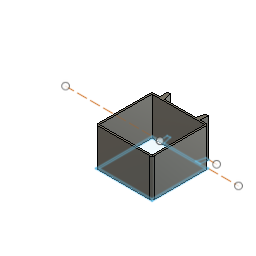
VoltmeterEnclosure (Autodesk Fusion 360 design; units mm, degrees)
Autodesk Fusion 360 part; units mm, degrees
note: some values were not read from the file. Set by a fixed rule: which sketch regions a step uses.
other "Base Mesh Feature1"
sketch "Sketch2" plane through (0, 0, 0) normal (0, 1, 0) x (1, 0, 0)
  line L0 (38.15, -96.15) -> (-38.15, -96.15)
  line L1 (-38.15, -96.15) -> (-38.15, -19.85)
  line L2 (-38.15, -19.85) -> (38.15, -19.85)
  line L3 (38.15, -19.85) -> (38.15, -96.15)
  line L4 (40.65, -98.65) -> (-40.65, -98.65)
  line L5 (-40.65, -98.65) -> (-40.65, -17.35)
  line L6 (-40.65, -17.35) -> (40.65, -17.35)
  line L7 (40.65, -17.35) -> (40.65, -98.65)
  line L8 (28.7422, -17.35) -> (22.7422, -17.35)
  line L9 (22.7422, -17.35) -> (25.6453, -5.7065)
  line L10 (22.7422, -17.35) -> (84.5269, -17.35) construction
  line L11 (30.0696, -6) -> (29.0766, -17.35)
  line L12 (30.0696, -6) -> (41.5439, -6) construction
  line L13 (28.7422, -17.35) -> (22.7422, -17.35)
  line L14 (30.0696, -6) -> (25.6453, -5.7065)
  line L15 (-22.8269, -17.5) -> (-25.7299, -5.8565)
  line L16 (-30, -6) -> (-25.7299, -5.8565)
  line L17 (-30, -6) -> (-28.9939, -17.5)
  line L18 (-22.8269, -17.5) -> (-165.8269, -17.35) construction
  line L19 (-28.8269, -17.5) -> (-22.8269, -17.5)
  dimension "d6" = -2.5
  dimension "d7" = 6
  dimension "d8" = 76
  dimension "d9" = 12
  dimension "d10" = 95
  constraint horizontal L0
  constraint vertical L1
  constraint horizontal L2
  constraint vertical L3
  constraint coincident L6 L8.start
  constraint parallel L6 L8
  constraint horizontal L10
  constraint horizontal L12
  constraint coincident L8 L11.end
  constraint symmetric L5 L10.end L18.end
  measures "d7" distance of L8.start L8.end
  measures "d8" angle of L9 L10
  measures "d9" distance of L8.end L9.end
  measures "d10" angle of L11 L12
extrude "Extrude1" add sketch "Sketch2" along normal blind 55 contours L6 L15 L16 L17
extrude "Extrude2" add sketch "Sketch2" along normal blind 55 contours L4 L5 L6 L7 L8 L13
extrude "Extrude3" add sketch "Sketch2" along normal blind 55 contours L6 L8 L9 L11 L13 L14
fillet "Fillet1" radius 3 1 edges at (40.65, 27.5, 98.65)
fillet "Fillet2" radius 3 1 edges at (-40.65, 27.5, 98.65)
fillet "Fillet3" radius 3 1 edges at (40.65, 27.5, 17.35)
fillet "Fillet4" radius 3 1 edges at (-40.65, 27.5, 17.35)
